Autodesk Fusion 360 part; units mm, degrees
(part 4 of 4)
equation "servo_connettore_larghezza = 7.0 mm" comment "Connettore SG90"
equation "servo_connettore_spessore = 3.0 mm" comment "Connettore SG90"
equation "passaggio_comune_larghezza = 9.0 mm" comment "Passaggio connettori SG90"
equation "passaggio_comune_lunghezza = 7.0 mm" comment "Passaggio connettori SG90"
equation "passaggio_arco_raggio = 28.0 mm" comment "Guida cavi azimut"
equation "passaggio_arco_larghezza = 9.0 mm" comment "Guida cavi azimut"
equation "ansa_azimut_lunghezza_libera = 210.0 mm" comment "Fascio ordinato nel canale"
equation "asola_fascetta_cavi_lunghezza = 5.0 mm" comment "Fermacavi torretta"
equation "asola_fascetta_cavi_larghezza = 2.0 mm" comment "Fermacavi torretta"
equation "asola_fascetta_cavi_interasse = 7.0 mm" comment "Fermacavi torretta"
equation "asola_fascetta_cannone_mobile_interasse = 12.0 mm" comment "Ancoraggio ansa elevazione"
equation "fermacavo_fisso_inferiore_larghezza = 18.0 mm" comment "Scarico trazione sotto uscita"
equation "fermacavo_fisso_inferiore_lunghezza = 12.0 mm" comment "Scarico trazione sotto uscita"
equation "fermacavo_fisso_inferiore_spessore = 2.0 mm" comment "Scarico trazione sotto uscita"
equation "fermacavo_fisso_asole_offset_x = 1.5 mm" comment "Sposta le asole fuori dal bordo anulare"
equation "fermacavo_fisso_ponte_larghezza = 20.0 mm" comment "Ponte strutturale verso il fondo anulare"
equation "fermacavo_fisso_ponte_lunghezza = 4.0 mm" comment "Ponte strutturale verso il fondo anulare"
equation "cannone_connettore_larghezza = 5.0 mm" comment "Connettore cannone"
equation "cannone_connettore_spessore = 3.0 mm" comment "Connettore cannone"
equation "cannone_passaggio_mobile_larghezza = 6.0 mm" comment "Passaggio sotto culla"
equation "cannone_passaggio_mobile_lunghezza = 4.0 mm" comment "Passaggio sotto culla"
equation "pcb_cannone_lunghezza = 50.0 mm" comment "PCB mobile cannone"
equation "pcb_cannone_larghezza = 50.0 mm" comment "PCB mobile cannone"
equation "pcb_cannone_spessore = 2.0 mm" comment "PCB mobile cannone"
equation "pcb_cannone_foro = 3.5 mm" comment "Fori PCB cannone"
equation "pcb_cannone_foro_bordo_x = 5.0 mm" comment "Fori PCB cannone"
equation "pcb_cannone_foro_bordo_y = 5.0 mm" comment "Fori PCB cannone"
equation "solenoide_diametro = 20.0 mm" comment "Zona solenoide"
equation "solenoide_lunghezza = 25.0 mm" comment "Zona solenoide"
equation "canna_diametro_esterno = 10.0 mm" comment "Canna tubolare"
equation "canna_diametro_interno = 8.0 mm" comment "Canna tubolare"
equation "canna_parete = 1.0 mm" comment "Canna tubolare"
equation "canna_sporgenza = 46.0 mm" comment "Canna tubolare"
equation "modulo_cannone_altezza = 23.0 mm" comment "Modulo mobile"
equation "culatta_proiettile_diametro_max_provvisorio = 7.0 mm" comment "Solo proiettile morbido e inerte"
equation "culatta_proiettile_lunghezza_max_provvisoria = 10.0 mm" comment "Ingombro di caricamento da verificare"
equation "culatta_guida_diametro_esterno = 11.0 mm" comment "Invito interno coassiale"
equation "culatta_guida_diametro_interno = 8.0 mm" comment "Invito interno coassiale"
equation "culatta_guida_lunghezza = 8.0 mm" comment "Invito interno coassiale"
equation "culatta_finestra_posteriore_larghezza = 14.0 mm" comment "Apertura a L removibile"
equation "culatta_asola_tetto_lunghezza = 12.0 mm" comment "Apertura a L removibile"
equation "culatta_coperchio_larghezza = 30.0 mm" comment "Coperchio a filo removibile"
equation "culatta_coperchio_lunghezza = 15.0 mm" comment "Coperchio a filo removibile"
equation "culatta_tasca_profondita = 2.0 mm" comment "Alloggiamento coperchio removibile"
equation "culatta_coperchio_spessore = 1.8 mm" comment "Coperchio a filo removibile"
equation "culatta_coperchio_gioco_verticale = 0.2 mm" comment "Coperchio leggermente ribassato"
equation "culatta_rinforzo_locale_spessore = 0.8 mm" comment "Rinforzo a U sotto la tasca"
equation "culatta_interasse_M2_5 = 21.5 mm" comment "Due viti accessibili dall'alto"
equation "culatta_foro_M2_5 = 2.7 mm" comment "Coperchio removibile"
equation "culatta_preforo_M2_5 = 2.2 mm" comment "Boss sotto il tetto"
equation "cannone_elevazione_min = -10.0 deg" comment "Limite proposto asse elevazione"
equation "cannone_elevazione_max = 35.0 deg" comment "Limite proposto asse elevazione"
equation "passaggio_arco_angolo_iniziale = 0.0 deg" comment "Inizio guida cavi di azimut"
equation "passaggio_arco_corsa = 360.0 deg" comment "Corsa totale guida cavi di azimut"
equation "torretta_azimut_min = -180.0 deg" comment "Limite software e giunto Fusion"
equation "torretta_azimut_max = 180.0 deg" comment "Limite software e giunto Fusion"
equation "d312 = cop_parete_altezza"
equation "d314 = cop_tetto_spessore"
equation "d332 = cop_parete_altezza"
equation "d338 = cop_tetto_spessore"
equation "d340 = cop_tetto_spessore"
equation "d342 = cop_tetto_spessore"
equation "d344 = cop_tetto_spessore"
equation "d348 = cop_tetto_spessore"
equation "d352 = cop_tetto_spessore"
equation "d356 = cop_tetto_spessore"
equation "d368 = cop_canale_fondo_spessore"
equation "d370 = cop_canale_fondo_spessore"
equation "d382 = cop_tetto_spessore"
equation "d416 = stepper_corpo_altezza"
equation "d424 = stepper_albero_lunghezza"
equation "d426 = stepper_albero_lunghezza"
equation "d430 = torre_base_spessore"
equation "d432 = torre_base_spessore"
equation "d434 = torre_base_spessore"
equation "d436 = torre_base_spessore"
equation "d444 = torre_base_spessore"
equation "d448 = torre_base_spessore"
equation "d452 = torre_base_spessore"
equation "d456 = torre_base_spessore"
equation "d460 = torre_base_spessore"
equation "d652 = servo_corpo_altezza"
equation "d668 = servo_corpo_altezza"
equation "d790 = pcb_cannone_spessore"
equation "d792 = pcb_cannone_spessore"
equation "d794 = pcb_cannone_spessore"
equation "d796 = pcb_cannone_spessore"
equation "d798 = pcb_cannone_spessore"
equation "d806 = solenoide_lunghezza"
equation "d810 = solenoide_lunghezza"
equation "d814 = canna_sporgenza"
equation "d818 = canna_sporgenza"
equation "guscio_torretta_parete = 2.5 mm" comment "Gusci removibili torretta"
equation "guscio_torretta_gioco = 0.5 mm" comment "Gioco attorno a telaio, servo e modulo mobile"
equation "guscio_cannone_foro_canna = 11.0 mm" comment "Passaggio canna nel guscio mobile"
named bodies: "Piano_inferiore_colonnine_M3_supporto_batteria_integrato", "Piano_superiore", "Guscio_laterale_continuo_166x176_Z0_Z76_griglie_fronte_retro", "Tetto_fisso_canale_cavi_guida_radiale_supporto_stepper_boss_M3", "Labbro_fisso_centraggio_radiale_torretta", "Rondella_assiale_DI76_DE94_spessore_0_8", "Corpo_stepper", "Albero_stepper", "Base_rotante_D100_sede_D_gola_guida_passaggio_cavi", "Piede_fermaglio_Est", "Piede_fermaglio_Ovest", "Piede_fermaglio_Nord", "Piede_fermaglio_Sud", "Base_parte_fissa", "Corpo_SG90_Sinistro", "Corpo_SG90_Destro", "Piastra_culla_mobile", "Albero_uscita_SG90_Sinistro", "Cornetto_croce_orizzontale_Sinistro", "Albero_uscita_SG90_Destro", "Cornetto_croce_orizzontale_Destro", "Disco_pieno_cornetto_Sinistra", "Mensola_sotto_culla_Sinistra", "Disco_pieno_cornetto_Destra", "Mensola_sotto_culla_Destra", "PCB_modulo_cannone_50x50", "Appoggio_solenoide_su_PCB", "Corpo_solenoide_riferimento", "Canna_tubolare_esterna", "Parete_posteriore_guscio_torretta", "Parete_esterna_carter_Sinistro", "Parete_esterna_carter_Destro", "Parete_mobile_Ovest", "Disco_pieno_cornetto_Sinistra (1)", "Disco_pieno_cornetto_Destra (1)", "Guida_interna_culatta_manuale", "Piastra_superiore_coperchio_culatta_a_filo"
